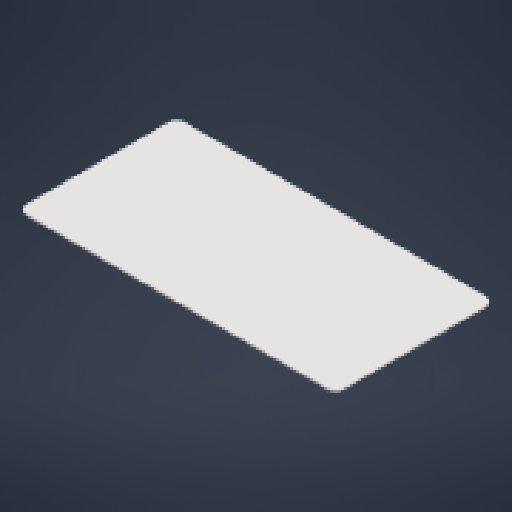
# Autodesk Inventor part: Bottom Cover
Saved by Autodesk Inventor 2023 (Build 270158000, 158)
## iProperties
Created: 2022-10-09
Part Number: Bottom Cover
Material: Stainless Steel
Document SubType Name: Modeling
Designer: Hilal Yahya
Density: 8 g/cm^3
Appearance: Semi-Polished
Author: Hilal Yahya
Autodesk Inventor part; units mm, degrees
ref_plane "YZ Plane" through (0, 0, 0) normal (1, 0, 0) x (0, 1, 0)
ref_plane "XZ Plane" through (0, 0, 0) normal (0, 1, 0) x (-1, 0, 0)
ref_plane "XY Plane" through (0, 0, 0) normal (0, 0, 1) x (1, 0, 0)
sketch "Sketch1" plane through (0, 0, 0) normal (0, 1, 0) x (-1, 0, 0)
  line L0 (-150, 100) -> (150, 100)
  line L1 (150, 100) -> (150, -100)
  line L2 (150, -100) -> (-150, -100)
  line L3 (-150, -100) -> (-150, 100)
  line L4 (-150, 100) -> (150, -100) construction
  line L5 (150, 100) -> (-150, -100) construction
  point P0 (0, 0)
  dimension "d0" = 300
  dimension "d1" = 200
  constraints: 12 end point, 2 midpoint, 2 parallel, 1 horizontal, 1 perpendicular
  measures "d0" distance of L1.end L2.end
  measures "d1" distance of L0.end L1.end
extrude "Extrusion1" add sketch "Sketch1" along normal blind 2
fillet "Fillet1" radius 10 4 edges at (150, 1, 100) (150, 1, -100) (-150, 1, -100) (-150, 1, 100)
body "Solid1"
